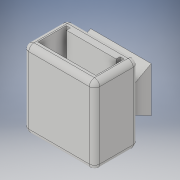
# Autodesk Inventor part: Schienenläufermitkeil_22.5
Saved by Autodesk Inventor 2018.3 (Build 223284000, 284)
## iProperties
Created: 2018-10-11
Part Number: Schienenläufermitkeil_22.5
Material: Generisch
Document SubType Name: Modeling
Designer: pgmadmin
Density: 1 g/cm^3
Appearance: Vorgabe
Author: pgmadmin
Autodesk Inventor part; units mm, degrees
ref_plane "YZ Plane" through (0, 0, 0) normal (1, 0, 0) x (0, 1, 0)
ref_plane "XZ Plane" through (0, 0, 0) normal (0, 1, 0) x (-1, 0, 0)
ref_plane "XY Plane" through (0, 0, 0) normal (0, 0, 1) x (1, 0, 0)
sketch "Skizze1" plane through (0, 0, 0) normal (0, 0, 1) x (1, 0, 0)
  line L0 (-14.1284, 0) -> (-14.1284, 11)
  line L1 (-14.1284, 11) -> (-12.5284, 11)
  line L2 (-12.5284, 11) -> (-12.5284, 1.6)
  line L3 (-12.5284, 1.6) -> (6.7716, 1.6)
  line L4 (6.7716, 1.6) -> (6.7716, 11)
  line L5 (6.7716, 11) -> (8.3716, 11)
  line L6 (8.3716, 11) -> (8.3716, 0)
  line L7 (8.3716, 0) -> (-14.1284, 0)
  line L8 (-16.6284, 14) -> (10.8716, 14)
  line L9 (10.8716, 14) -> (10.8716, -3)
  line L10 (10.8716, -3) -> (-16.6284, -3)
  line L11 (-16.6284, -3) -> (-16.6284, 14)
  line L12 (-12.5284, 9.5) -> (6.7716, 9.5)
  point P0 (0, 0)
  dimension "d0" = 11
  dimension "d1" = 1.6
  dimension "d2" = 19.3
  dimension "d3" = 1.6
  dimension "d4" = 1.6
  dimension "d5" = 3
  dimension "d6" = 3
  dimension "d7" = 2.5
  dimension "d8" = 2.5
  dimension "d9" = 1.5
  constraints: 26 end point, 8 perpendicular, 4 point on line, 2 parallel, 1 horizontal, 1 vertical
  measures "d0" distance of L0.start L0.end
  measures "d1" distance of L0.end L1.end
  measures "d2" distance of L2.end L3.end
  measures "d3" distance of L4.end L5.end
  measures "d4" distance between parallel lines of L3 L7
  measures "d5" distance between parallel lines of L10 L7
  measures "d6" distance between parallel lines of L8 L1
  measures "d7" distance between parallel lines of L11 L0
  measures "d8" distance between parallel lines of L9 L6
  measures "d9" distance of L1.end L12.start
extrude "Extrusion1" add sketch "Skizze1" along normal blind 30
fillet "Rundung1" radius 2 12 edges at (10.8716, 14, 15) (10.8716, -3, 15) (-16.6284, -3, 15) (-16.6284, 14, 15) (-2.8784, 14, 30) (-16.6284, 5.5, 30) (-2.8784, -3, 30) (10.8716, 5.5, 30) (10.8716, 5.5, 0) (-2.8784, -3, 0) (-2.8784, 14, 0) (-16.6284, 5.5, 0)
sketch "Skizze2" plane through (10.8716, -1, 28) normal (1, 0, 0) x (0, 0, -1)
  line L0 (0, 15) -> (26, 15) projected
  line L1 (8, 15) -> (4.25, 22)
  line L2 (4.25, 22) -> (21.75, 22)
  line L3 (21.75, 22) -> (18, 15)
  line L4 (28, 0) -> (28, 13) projected
  point P0 (28, 1)
  dimension "d13" = 10
  dimension "d15" = 7
  dimension "d16" = 3.75
  dimension "d17" = 3.75
  dimension "d18" = 17.5
  dimension "d19" = 10
  constraints: 6 end point, 2 point on line, 1 parallel
  measures "d13" distance of L3.end L1.start
  measures "d15" vertical distance of L1.end L1.start
  measures "d16" horizontal distance of L2.end L3.end
  measures "d17" horizontal distance of L1.start L1.end
  measures "d18" distance of L1.end L2.end
  measures "d19" distance from line of L4 L3.end
extrude "Extrusion2" add sketch "Skizze2" against normal blind 27.5
sketch "Skizze4" plane through (10.8716, 21, 23.75) normal (0, 1, 0) x (1, 0, 0)
  line L0 (-25.5, 21.75) -> (-25.5, -4.25) projected
  line L1 (-27.5, 3.75) -> (-27.5, 0) projected
  line L2 (-25.5, 17.5243) -> (-27.5, 17.5243)
  line L3 (-27.5, 17.5243) -> (-27.5, 0)
  line L4 (-27.5, 0) -> (-25.5, 0)
  line L5 (-25.5, 0) -> (-25.5, 17.5243)
  line L6 (0, 17.5) -> (-27.5, 17.5) projected
  line L7 (-2, 3.75) -> (-2, -4.25) projected
  line L8 (0, 17.5) -> (-2, 17.5)
  line L9 (-2, 17.5) -> (-2, 0)
  line L10 (-2, 0) -> (0, 0)
  line L11 (0, 0) -> (0, 17.5)
  point P0 (-10.8716, 23.75)
  constraints: 16 end point, 4 parallel, 3 point on line, 2 horizontal, 2 perpendicular
extrude "Extrusion4" cut sketch "Skizze4" against normal blind 7
